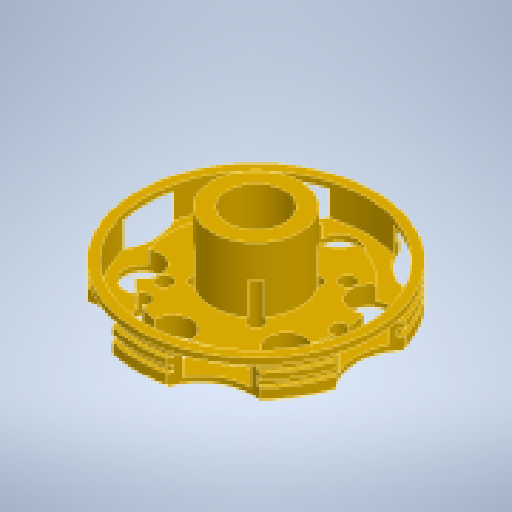
# Autodesk Inventor part: BASE
Saved by Autodesk Inventor 2023.1 (Build 271208000, 208)
## iProperties
Created: 2022-10-25
Part Number: BASE
Material: Aluminum 6061
Document SubType Name: Modeling
Designer: Nathan Cai
Density: 2.7 g/cm^3
Appearance: Gold
Author: Nathan Cai
Autodesk Inventor part; units mm, degrees
ref_plane "YZ Plane" through (0, 0, 0) normal (1, 0, 0) x (0, 1, 0)
ref_plane "XZ Plane" through (0, 0, 0) normal (0, 1, 0) x (-1, 0, 0)
ref_plane "XY Plane" through (0, 0, 0) normal (0, 0, 1) x (1, 0, 0)
sketch "Sketch1" plane through (0, 0, 0) normal (0, 0, 1) x (1, 0, 0)
  line L0 (0, 0) -> (23, 0)
  line L1 (23, 0) -> (23, 7.5)
  line L2 (23, 7.5) -> (0, 7.5) construction
  line L3 (0, 7.5) -> (0, 0)
  line L4 (0, 7.5) -> (21.25, 7.5) construction
  line L5 (21.25, 7.5) -> (21.25, 1.35)
  line L6 (21.25, 1.35) -> (0, 1.35)
  line L7 (0, 1.35) -> (0, 7.5)
  line L8 (21.25, 7.5) -> (23, 7.5)
  line L9 (22.25, 6.25) -> (23.75, 6.25)
  line L10 (23.75, 6.25) -> (23.75, 5)
  line L11 (23.75, 5) -> (22.25, 5)
  line L12 (22.25, 5) -> (22.25, 6.25)
  line L13 (22.25, 6.25) -> (23.75, 5) construction
  line L14 (23.75, 6.25) -> (22.25, 5) construction
  line L15 (22.25, 2.5) -> (22.25, 3.75)
  line L16 (22.25, 3.75) -> (23.75, 3.75)
  line L17 (23.75, 3.75) -> (23.75, 2.5)
  line L18 (23.75, 2.5) -> (22.25, 2.5)
  line L19 (22.25, 3.75) -> (23.75, 2.5) construction
  line L20 (23.75, 3.75) -> (22.25, 2.5) construction
  line L21 (0, 0) -> (16.5, 0)
  line L22 (16.5, 0) -> (16.5, 4)
  line L23 (16.5, 4) -> (0, 4)
  line L24 (0, 4) -> (0, 0)
  line L25 (0, 0) -> (5.5, 0)
  line L26 (5.5, 0) -> (5.5, 16.5)
  line L27 (5.5, 16.5) -> (0, 16.5)
  line L28 (0, 16.5) -> (0, 0)
  line L29 (0, 0) -> (8.5, 0)
  line L30 (8.5, 0) -> (8.5, 16.5)
  line L31 (8.5, 16.5) -> (0, 16.5)
  line L32 (0, 16.5) -> (0, 0)
  point P0 (23, 5.625)
  point P1 (23, 3.125)
  point P2 (16.5, 1.35)
  point P3 (8.5, 4)
  point P4 (23, 2.5)
  point P5 (23, 3.75)
  point P6 (23, 5)
  point P7 (23, 6.25)
  dimension "d0" = 23
  dimension "d1" = 7.5
  dimension "d2" = 1.35
  dimension "d3" = 1.75
  dimension "d4" = 1.5
  dimension "d5" = 1.25
  dimension "d6" = 1.25
  dimension "d9" = 2.5
  dimension "d14" = 16.5
  dimension "d15" = 4
  dimension "d16" = 5.5
  dimension "d17" = 16.5
  dimension "d18" = 8.5
  constraints: 66 end point, 12 parallel, 7 horizontal, 6 perpendicular, 2 midpoint, 2 point on line, 1 vertical, 11 other
  measures "d0" distance of L2.end L1.end
  measures "d1" distance of L1.end L0.end
  measures "d2" distance between parallel lines of L0 L6
  measures "d3" distance between parallel lines of L1 L5
  measures "d4" distance of L10.end L11.end
  measures "d5" distance of L9.end L10.end
  measures "d6" distance between parallel lines of L2 L9
  measures "d9" distance of L9.start L15.end
  measures "d14" distance of L23.end L22.end
  measures "d15" distance of L22.end L21.end
  measures "d16" distance of L27.end L26.end
  measures "d17" distance of L26.end L25.end
  measures "d18" distance of L31.end L30.end
revolve "Revolution1" add sketch "Sketch1" angle 360 about axis through (0, 16.5, 0) along (0, -1, 0) contours L26 L6 L30 L0 | L30 L6 L22 L0 | L26 L23 L30 L6 | L22 L6 L5 L8 L1 L9 L12 L11 L16 L15 L18 L0 | L30 L23 L22 L6 | L26 L31 L30 L23
sketch "Sketch2" plane through (0, 0, 0) normal (0, -1, 0) x (1, 0, 0)
  circle A0 centre (0, 0) radius 5.5
  circle A1 centre (0, 0) radius 16 construction
  circle A2 centre (0, 16) radius 3.5
  line L0 (0, 0) -> (0, 23) construction
  circle A3 centre (0, 0) radius 23 construction
  line L1 (0, 0) -> (11.5, 19.918584) construction
  circle A4 centre (0, 0) radius 19.5 construction
  circle A5 centre (14.75, 25.547749) radius 10
  circle A6 centre (0, 0) radius 8 construction
  circle A7 centre (0, 0) radius 9.5 construction
  circle A8 centre (0, 0) radius 12.5 construction
  circle A9 centre (0, 0) radius 8.5 construction
  line L2 (0, 0) -> (6.717514, 6.717514) construction
  line L3 (0, 0) -> (-8.838835, 8.838835) construction
  circle A10 centre (6.717514, 6.717514) radius 1.5
  circle A11 centre (-5.656854, 5.656854) radius 1.5
  circle A12 centre (-8.838835, 8.838835) radius 1.5
  circle A13 centre (8.838835, -8.838835) radius 1.5
  circle A14 centre (5.656854, -5.656854) radius 1.5
  circle A15 centre (-6.717514, -6.717514) radius 1.5
  circle A16 centre (-14.75, 25.547749) radius 10
  circle A17 centre (-13.856406, 8) radius 3.5
  circle A18 centre (-29.5, 0) radius 10
  circle A19 centre (-13.856406, -8) radius 3.5
  circle A20 centre (-14.75, -25.547749) radius 10
  circle A21 centre (0, -16) radius 3.5
  circle A22 centre (14.75, -25.547749) radius 10
  circle A23 centre (13.856406, -8) radius 3.5
  circle A24 centre (29.5, 0) radius 10
  circle A25 centre (13.856406, 8) radius 3.5
  line L4 (0, 0) -> (23, 0) construction
  circle A26 centre (0, 0) radius 15.75 construction
  line L5 (-8, 13.856406) -> (16, 0) construction
  line L6 (16, 0) -> (-8, -13.856406) construction
  line L7 (-8, -13.856406) -> (-8, 13.856406) construction
  line L8 (-8, 13.856406) -> (0, 0) construction
  circle A27 centre (-8, 13.856406) radius 1.5
  circle A28 centre (-8, -13.856406) radius 1.5
  circle A29 centre (16, 0) radius 1.5
  line L9 (30.047434, 5.875) -> (15.952566, 5.875)
  line L10 (15.952566, 5.875) -> (15.952566, -5.875) construction
  line L11 (15.952566, -5.875) -> (30.047434, -5.875)
  line L12 (30.047434, -5.875) -> (30.047434, 5.875)
  line L13 (30.047434, 5.875) -> (15.952566, -5.875) construction
  line L14 (15.952566, 5.875) -> (30.047434, -5.875) construction
  circle A30 centre (0, 0) radius 17
  line L15 (29.5, 0) -> (0, 0) construction
  arc A31 (16.642692, -3.467105) -> (18.600655, -5.875) centre (18.600655, -3.875) ccw
  arc A32 (18.600655, 5.875) -> (16.642692, 3.467105) centre (18.600655, 3.875) ccw
  point P0 (18.600655, 5.875)
  point P1 (16.642692, 3.467105)
  dimension "d25" = 16
  dimension "d26" = 19
  dimension "d27" = 25
  dimension "d20" = 32
  dimension "d21" = 7
  dimension "d22" = 30
  dimension "d23" = 39
  dimension "d24" = 20
  dimension "d28" = 45
  dimension "d30" = 3
  dimension "d31" = 3
  dimension "d32" = 3
  dimension "d35" = 360
  dimension "d39" = 360
  dimension "d41" = 31.5
  dimension "d42" = 30
  dimension "d43" = 3
  dimension "d46" = 360
  dimension "d58" = 11.75
  dimension "d59" = 34
  dimension "d60" = 4
  constraints: 32 end point, 27 centre point, 11 coincident, 11 point on circle, 5 point on line, 3 symmetric about line, 3 tangent, 2 midpoint, 2 parallel, 2 perpendicular, 1 horizontal, 1 vertical, 62 other
  measures "d20" diameter of A1
  measures "d21" diameter of A2
  measures "d22" angle of L0 L1
  measures "d23" diameter of A4
  measures "d24" diameter of A5
  measures "d28" angle of L0 L2
  measures "d30" diameter of A10
  measures "d31" diameter of A11
  measures "d32" diameter of A12
  measures "d41" diameter of A26
  measures "d42" angle of L0 L8
  measures "d43" diameter of A27
  measures "d58" distance of L10.end L9.end
  measures "d59" diameter of A30
  measures "d60" diameter of A31
chamfer "Chamfer1" distance 0.5 angle 45 1 edges at (-23, 0, 0)
extrude "Extrusion1" cut sketch "Sketch2" against normal blind 6.25 contours A32 L9 A24 L11 A31 A30 A29 | A29 A30 | L9 L12 L11 A24 | A5 | A16 | A18 | A20 | A22 picked at (17.153291, -0.236627) picked at (26.531623, 0)
extrude "Extrusion2" cut sketch "Sketch2" against normal blind 10 contours A0 | A2 A30 | A30 A2 | A30 A25 | A25 L9 A30 | A30 A27 | A27 A30 | A30 L9 A25 | A30 A17 | A17 A30 | A30 A19 | A19 A30 | A30 A23 | A23 L11 A30 | A30 A28 | A28 A30 | A23 A30 L11 | A30 A21 | A21 A30 | A10 | A11 | A12 | A13 | A14 | A15
chamfer "Chamfer2" distance 0.25 angle 45 25 edges at (9.75, 0, 16.8875) (9.75, 0, -16.8875) (-9.75, 0, -16.8875) (-19.5, 0, 0) (-9.75, 0, 16.8875) (-3.5, 0, 16) (5.2175, 0, 6.7175) (10.3564, 0, 8) (10.3564, 0, -8) (7.3388, 0, -8.8388) (4.1569, 0, -5.6569) (-3.5, 0, -16) (-8.2175, 0, -6.7175) (-9.5, 0, -13.8564) (-17.3564, 0, -8) (-17.3564, 0, 8) (-10.3388, 0, 8.8388) (-9.5, 0, 13.8564) (-7.1569, 0, 5.6569) (-5.5, 0, 0) (17.0489, 0, -5.1368) (17, 0, 0) (17.0489, 0, 5.1368) (20.1601, 0, 5.875) (20.1601, 0, -5.875)
body "Solid1"
